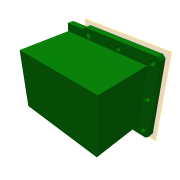
# Autodesk Inventor part: cellSTORM_v5_cellphonestage
Saved by Autodesk Inventor 2019 (Build 230136000, 136)
## iProperties
Created: 2020-04-25
Part Number: cellSTORM_v5_cellphonestage
Material: Generic
Document SubType Name: Modeling
Designer: diederichbenedict
Density: 1 g/cm^3
Appearance: Dark Green
Author: diederichbenedict
Autodesk Inventor part; units mm, degrees
ref_plane "YZ Plane" through (0, 0, 0) normal (1, 0, 0) x (0, 1, 0)
ref_plane "XZ Plane" through (0, 0, 0) normal (0, 1, 0) x (-1, 0, 0)
ref_plane "XY Plane" through (0, 0, 0) normal (0, 0, 1) x (1, 0, 0)
ref_plane "Work Plane1" through (0, 0, 0) normal (0, 0, 1) x (1, 0, 0)
sketch "Sketch1" plane through (0, 0, 0) normal (0, 0, 1) x (1, 0, 0)
  circle A0 centre (25, 25) radius 1.95 projected
  circle A1 centre (25, 0) radius 1.95 projected
  circle A2 centre (0, 25) radius 1.95 projected
  circle A3 centre (-25, 0) radius 1.95 projected
  circle A4 centre (-25, -25) radius 1.95 projected
  circle A5 centre (25, 25) radius 1.95 projected
  circle A6 centre (25, -25) radius 1.95 projected
  circle A7 centre (-25, 25) radius 1.95 projected
  circle A8 centre (25, 0) radius 1.95 projected
  circle A9 centre (0, -25) radius 1.95 projected
  line L0 (-28, 30) -> (-30, 28) projected
  line L1 (-30, 28) -> (-30, -28) projected
  line L2 (-30, -28) -> (-28, -30) projected
  line L3 (-28, -30) -> (28, -30) projected
  line L4 (28, -30) -> (30, -28) projected
  line L5 (30, -28) -> (30, 28) projected
  line L6 (30, 28) -> (28, 30) projected
  line L7 (28, 30) -> (-28, 30) projected
  point P0 (0, 0)
extrude "Extrusion1" add sketch "Sketch1" along normal blind 5
sketch "Sketch2" plane through (0, 0, 5) normal (0, 0, 1) x (1, 0, 0)
  circle A0 centre (0, -25) radius 1.95 projected
  circle A1 centre (-25, 25) radius 1.95 projected
  circle A2 centre (25, -25) radius 1.95 projected
  circle A3 centre (-25, -25) radius 1.95 projected
  circle A4 centre (-25, 0) radius 1.95 projected
  circle A5 centre (0, 25) radius 1.95 projected
  circle A6 centre (25, 0) radius 1.95 projected
  circle A7 centre (25, 25) radius 1.95 projected
  line L0 (-28, 30) -> (-30, 28) projected
  line L1 (-30, 28) -> (-30, -28) projected
  line L2 (-30, -28) -> (-28, -30) projected
  line L3 (-28, -30) -> (28, -30) projected
  line L4 (28, -30) -> (30, -28) projected
  line L5 (30, -28) -> (30, 28) projected
  line L6 (30, 28) -> (28, 30) projected
  line L7 (28, 30) -> (-28, 30) projected
  line L8 (-30, 28) -> (-30, -28) projected
  line L9 (-30, -22) -> (22, -22)
  line L10 (22, -22) -> (22, 22)
  line L11 (22, 22) -> (-30, 22)
  line L12 (-30, 22) -> (-30, -22)
  point P0 (0, 0)
  dimension "d2" = 8
  dimension "d3" = 8
  dimension "d4" = 8
  constraints: 8 end point, 2 parallel, 1 horizontal, 1 perpendicular, 1 point on line
  measures "d2" distance between parallel lines of L9 L3
  measures "d3" distance between parallel lines of L7 L11
  measures "d4" distance between parallel lines of L5 L10
ref_plane "Work Plane2" through (-93.15, -42.6288, 31.9788) normal (0, 0, -1) x (0, 1, 0)
extrude "Extrusion2" add sketch "Sketch2" along normal blind 40 contours A4 | L11 L10 L9 L1
sketch "Sketch3" plane through (-30, -28, 0) normal (-1, 0, 0) x (0, 0, 1)
  line L0 (0, 56) -> (0, 0) projected
  line L1 (0, 0) -> (5, 0) projected
  line L2 (5, 6) -> (5, 0) projected
  line L3 (5, 6) -> (45, 6) projected
  line L4 (5, 50) -> (45, 50) projected
  line L5 (5, 56) -> (5, 50) projected
  line L6 (0, 56) -> (5, 56) projected
  line L7 (45, 50) -> (45, 6) projected
  point P0 (0, 28)
extrude "Extrusion3" add sketch "Sketch3" along normal blind 10
sketch "Sketch4" plane through (22, -22, 0) normal (0, 0, 1) x (1, 0, 0)
  line L0 (-62, 0) -> (0, 0) projected
  line L1 (0, 44) -> (-62, 44) projected
  line L2 (-62, 0) -> (-62, 44) projected
  arc A0 (-111.65, 45.2512) -> (-115.15, 41.7512) centre (-111.65, 41.7512) ccw projected
  line L3 (-115.15, -17.1288) -> (-115.15, 41.7512) projected
  arc A1 (-115.15, -17.1288) -> (-111.65, -20.6288) centre (-111.65, -17.1288) ccw projected
  line L4 (28.35, -20.6288) -> (-111.65, -20.6288) projected
  arc A2 (28.35, -20.6288) -> (31.85, -17.1288) centre (28.35, -17.1288) ccw projected
  line L5 (31.85, 41.7512) -> (31.85, -17.1288) projected
  arc A3 (31.85, 41.7512) -> (28.35, 45.2512) centre (28.35, 41.7512) ccw projected
  line L6 (-111.65, 45.2512) -> (28.35, 45.2512) projected
  line L7 (0, 0) -> (0, 44) projected
  line L8 (-62, 44) -> (0, 44)
  line L9 (0, 44) -> (0, 0)
  line L10 (0, 0) -> (-62, 0)
  line L11 (-62, 0) -> (-62, 44)
  line L12 (-5, 39) -> (-57, 39)
  line L13 (-57, 39) -> (-57, 5)
  line L14 (-57, 5) -> (-5, 5)
  line L15 (-5, 5) -> (-5, 39)
  point P0 (-22, 22)
  dimension "d9" = 5
  constraints: 16 end point, 4 parallel, 2 perpendicular, 1 horizontal, 3 other
  measures "d9" distance between parallel lines of L8 L12
extrude "Extrusion4" cut sketch "Sketch4" along normal blind 40 contours L15 L14 L13 L12
sketch "Sketch6" plane through (-40, -28, 0) normal (-1, 0, 0) x (0, 0, 1)
  line L0 (0, 56) -> (0, 0) projected
  line L1 (0, 0) -> (5, 0) projected
  line L2 (5, 0) -> (5, 6) projected
  line L3 (5, 6) -> (45, 6) projected
  line L4 (45, 50) -> (5, 50) projected
  line L5 (5, 50) -> (5, 56) projected
  line L6 (5, 56) -> (0, 56) projected
  line L7 (45, 6) -> (45, 50) projected
  point P0 (0, 28)
extrude "Extrusion6" add sketch "Sketch6" along normal blind 5
sketch "Sketch7" plane through (-45, -28, 0) normal (-1, 0, 0) x (0, 0, 1)
  circle A0 centre (41, 25.7717) radius 1.45 projected
  circle A1 centre (23.9, 21.2512) radius 1.45 projected
  circle A2 centre (3.3174, 32.2512) radius 1.45 projected
  circle A3 centre (3.3174, 53) radius 1.45 projected
  line L0 (40, 45) -> (40, 11) projected
  circle A4 centre (41, 8.1883) radius 1.45 projected
  circle A5 centre (4.9143, 21.2512) radius 1.45 projected
  circle A6 centre (23.9337, 3.5995) radius 1.45 projected
  circle A7 centre (41, 25.7717) radius 1.45 projected
  circle A8 centre (41.0502, 56) radius 1.45 projected
  circle A9 centre (41, 0.7395) radius 1.45 projected
  circle A10 centre (23.9, 21.2512) radius 1.45 projected
  circle A11 centre (23.9, 13.4229) radius 1.45 projected
  circle A12 centre (41, 43.0063) radius 1.45 projected
  line L1 (37.1004, -11.7636) -> (45, -11.7636) projected
  line L2 (45, -11.7636) -> (45, 58) projected
  line L3 (26.9, 58) -> (26.9, 25.2512) projected
  line L4 (26.9, 25.2512) -> (-10.2763, 25.2512) projected
  line L5 (-10.2763, 25.2512) -> (37.1004, -11.7636) projected
  line L6 (45, 58) -> (26.9, 58) projected
  point P0 (0, 28)
  point P1 (4.6577, 21.4172)
hole "Hole1" at (-45, 15.0063, 41) at (-45, -2.2283, 41) at (-45, -19.8117, 41) at (-45, -14.5771, 23.9) at (-45, -6.7488, 23.9) at (-45, 4.2512, 3.3174) at (-45, 25, 3.3174) at (-45, -6.7488, 4.9143) direction (1, 0, 0) diameter 2.9 depth 20 tip angle 118
pattern_linear "Rectangular Pattern1" count 4 spacing 4 along (0, 0, -1) of "Hole1"
body "Solid1"
